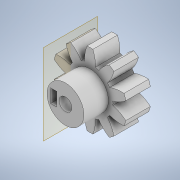
# Autodesk Inventor part: Gear1
Saved by Autodesk Inventor 2020 (Build 240168000, 168)
## iProperties
Created: 2020-09-23
Part Number: Gear1
Material: Generic
Document SubType Name: Modeling
Designer: s4393944
Density: 1 g/cm^3
Appearance: Default
Author: s4393944
Autodesk Inventor part; units mm, degrees
ref_plane "XZ Plane" through (0, 0, 0) normal (0, 1, 0) x (-1, 0, 0)
ref_plane "XY Plane" through (0, 0, 0) normal (0, 0, 1) x (1, 0, 0)
sketch "Sketch1" plane through (0, 0, 0) normal (0, 0, 1) x (1, 0, 0)
  circle A0 centre (0, 0) radius 25
  dimension "d2" = 50
  constraints: 1 centre point, 1 coincident
  measures "d2" diameter of A0
extrude "Extrusion1" add sketch "Sketch1" along normal blind 10
spur gear teeth "Spur Gear1" teeth 10 pitch diameter 25 tip diameter 30 root diameter 18.75 face width 20 trims to tip circle yes start plane through (0, 0, 10) normal (0, 0, 1) x (1, 0, 0)
sketch "Sketch2" plane through (0, 0, 10) normal (0, 0, 1) x (1, 0, 0)
  circle A0 centre (0, 0) radius 7.5
  dimension "d3" = 15
  constraints: 1 centre point, 1 coincident
  measures "d3" diameter of A0
extrude "Extrusion2" add sketch "Sketch2" along normal blind 10
sketch "Sketch3" plane through (0, 0, 20) normal (0, 0, 1) x (1, 0, 0)
  circle A0 centre (0, 0) radius 2.6
  dimension "d6" = 5.2
  constraints: 1 centre point, 1 coincident
  measures "d6" diameter of A0
extrude "Extrusion3" cut sketch "Sketch3" against normal up to surface (20 mm away)
ref_plane "Work Plane1" through (-7.9375, 0, 0) normal (1, 0, 0) x (0, 1, 0)
sketch "Sketch5" plane through (-7.9375, 0, 0) normal (1, 0, 0) x (0, 1, 0)
  circle A0 centre (0, 15) radius 1.5
  point P0 (0, 0)
  dimension "d12" = 3
  dimension "d13" = 15
  constraints: 1 centre point
  measures "d12" diameter of A0
  measures "d13" distance of point (0, 0) A0.centre
extrude "Extrusion5" cut sketch "Sketch5" along normal up to next
sketch "Sketch6" plane through (0, 0, 20) normal (0, 0, 1) x (1, 0, 0)
  line L0 (-6.0479, 2.75) -> (-3.5479, 2.75)
  line L1 (-3.5479, 2.75) -> (-3.5479, -2.75)
  line L2 (-3.5479, -2.75) -> (-6.0479, -2.75)
  line L3 (-6.0479, -2.75) -> (-6.0479, 2.75)
  line L4 (-6.0479, 2.75) -> (-3.5479, -2.75) construction
  line L5 (-3.5479, 2.75) -> (-6.0479, -2.75) construction
  point P0 (0, 0)
  point P1 (-4.7979, 0)
  dimension "d17" = 2.5
  dimension "d19" = 2.75
  dimension "d20" = 5.5
  constraints: 12 end point, 2 midpoint, 2 parallel, 1 horizontal, 1 perpendicular
  measures "d17" distance of L0.start L0.end
  measures "d19" distance from line of point (0, 0) L2
  measures "d20" distance of L2.end L0.start
extrude "Extrusion6" cut sketch "Sketch6" against normal blind 7.5
body "Solid1"
